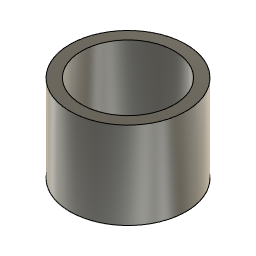
сборка с лопаткой v2 (Autodesk Fusion 360 archive; units mm, degrees)
design "подставки под нагреватель"
Autodesk Fusion 360 part; units mm, degrees
sketch "Sketch1" plane through (0, 0, 0) normal (0, 0, 1) x (1, 0, 0)
  circle A0 centre (0, 0) radius 10
  circle A1 centre (0, 0) radius 8
  dimension "d1" = 20
  dimension "d2" = 16
  constraint coincident A0.centre A1.centre
  constraint concentric A0 A1
  measures "d1" diameter of A0
  measures "d2" diameter of A1
extrude "Extrude1" add sketch "Sketch1" along normal blind 15

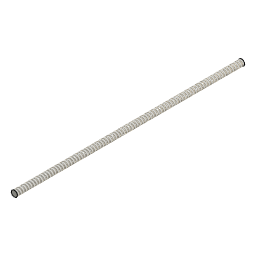
design "винт"
Autodesk Fusion 360 part; units mm, degrees
sketch "Sketch1" plane through (0, 0, 0) normal (0, 1, 0) x (1, 0, 0)
  circle A0 centre (0, 0) radius 4
  dimension "d1" = 8
  constraint coincident A0.centre origin
  measures "d1" diameter of A0
extrude "Extrude1" add sketch "Sketch1" along normal blind 300
thread "Thread1" "GOST Self-tapping Screw Thread 8.0 M8x3.5 h13" major diameter 7.89 minor diameter 5.51 pitch 3.5 angle 60 resizes the face on face at (3.995, 200, 0.1994)

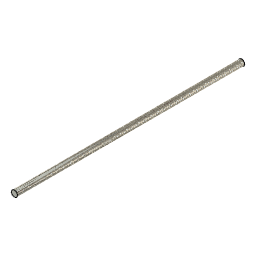
design "вал"
Autodesk Fusion 360 part; units mm, degrees
sketch "Sketch1" plane through (0, 0, 0) normal (0, 1, 0) x (1, 0, 0)
  circle A0 centre (0, 0) radius 4
  dimension "d1" = 8
  constraint coincident A0.centre origin
  measures "d1" diameter of A0
extrude "Extrude1" add sketch "Sketch1" along normal blind 300

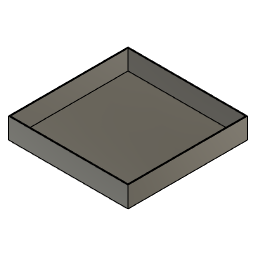
design "ванна"
Autodesk Fusion 360 part; units mm, degrees
sketch "Sketch1" plane through (0, 0, 0) normal (0, 0, 1) x (1, 0, 0)
  line L0 (122.5, 122.5) -> (-122.5, 122.5)
  line L1 (-122.5, 122.5) -> (-122.5, -122.5)
  line L2 (-122.5, -122.5) -> (122.5, -122.5)
  line L3 (122.5, -122.5) -> (122.5, 122.5)
  line L4 (122.5, 122.5) -> (-122.5, -122.5) construction
  line L5 (-122.5, 122.5) -> (122.5, -122.5) construction
  line L6 (120.5, 120.5) -> (-120.5, 120.5)
  line L7 (-120.5, 120.5) -> (-120.5, -120.5)
  line L8 (-120.5, -120.5) -> (120.5, -120.5)
  line L9 (120.5, -120.5) -> (120.5, 120.5)
  line L10 (120.5, 120.5) -> (-120.5, -120.5) construction
  line L11 (-120.5, 120.5) -> (120.5, -120.5) construction
  dimension "d1" = 245
  dimension "d2" = 245
  dimension "d3" = 241
  dimension "d4" = 241
  constraint horizontal L0
  constraint perpendicular L0 L1
  constraint parallel L0 L2
  constraint parallel L1 L3
  constraint coincident L4 origin
  constraint coincident L5 origin
  constraint horizontal L6
  constraint perpendicular L6 L7
  constraint parallel L6 L8
  constraint parallel L7 L9
  constraint coincident L10 origin
  constraint coincident L11 origin
  measures "d1" distance of L0.end L1.end
  measures "d2" distance of L1.end L2.end
  measures "d3" distance of L7.end L8.end
  measures "d4" distance of L6.end L7.end
extrude "Extrude1" add sketch "Sketch1" along normal blind 42.5
extrude "Extrude2" add sketch "Sketch1" along normal blind 2 contours L6 L7 L8 L9

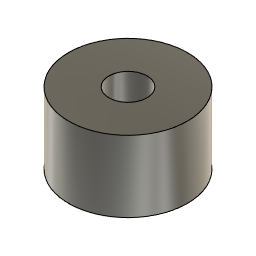
design "ножка"
Autodesk Fusion 360 part; units mm, degrees
sketch "Sketch1" plane through (0, 0, 0) normal (0, 0, 1) x (1, 0, 0)
  circle A0 centre (0, 0) radius 12.5
  circle A1 centre (0, 0) radius 4
  dimension "d1" = 25
  dimension "d2" = 8
  constraint coincident A0.centre A1.centre
  measures "d1" diameter of A0
  measures "d2" diameter of A1
extrude "Extrude1" add sketch "Sketch1" along normal blind 15

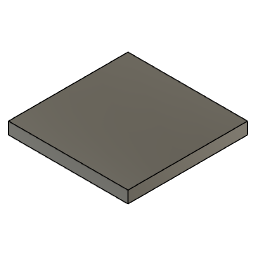
design "нагреватель"
Autodesk Fusion 360 part; units mm, degrees
sketch "Sketch1" plane through (0, 0, 0) normal (0, 0, 1) x (1, 0, 0)
  line L0 (150, 150) -> (-150, 150)
  line L1 (-150, 150) -> (-150, -150)
  line L2 (-150, -150) -> (150, -150)
  line L3 (150, -150) -> (150, 150)
  line L4 (150, 150) -> (-150, -150) construction
  line L5 (-150, 150) -> (150, -150) construction
  dimension "d1" = 300
  dimension "d2" = 300
  constraint horizontal L0
  constraint perpendicular L0 L1
  constraint parallel L0 L2
  constraint parallel L1 L3
  constraint coincident L4 origin
  constraint coincident L5 origin
  measures "d1" distance of L1.end L2.end
  measures "d2" distance of L0.end L1.end
extrude "Extrude1" add sketch "Sketch1" along normal blind 30
